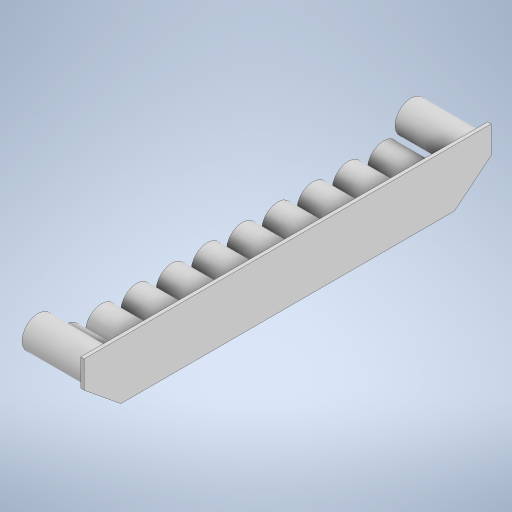
# Autodesk Inventor part: Enemy_Track_inertia
Saved by Autodesk Inventor 2024 (Build 280153000, 153)
## iProperties
Created: 2026-05-21
Part Number: Enemy_Track_inertia
Material: Generic
Document SubType Name: Modeling
Designer: warny
Density: 1 g/cm^3
Appearance: Default
Author: warny
Autodesk Inventor part; units mm, degrees
ref_plane "YZ Plane" through (0, 0, 0) normal (1, 0, 0) x (0, 1, 0)
ref_plane "XZ Plane" through (0, 0, 0) normal (0, 1, 0) x (-1, 0, 0)
ref_plane "XY Plane" through (0, 0, 0) normal (0, 0, 1) x (1, 0, 0)
sketch "Sketch1" plane through (0, 0, 0) normal (1, 0, 0) x (0, 1, 0)
  line L0 (66.79, 404) -> (66.79, -404)
  line L1 (66.79, -404) -> (12.72, -404)
  line L2 (12.72, -404) -> (-46.497, -331.3)
  line L3 (-46.497, -331.3) -> (-46.497, 331.3)
  line L4 (-46.497, 331.3) -> (12.72, 404)
  line L5 (12.72, 404) -> (66.79, 404)
  point P0 (0, 0)
  dimension "d0" = 331.3
  dimension "d1" = 331.3
  dimension "d2" = 46.497
  dimension "d3" = 46.497
  dimension "d4" = 12.72
  dimension "d5" = 12.72
  dimension "d6" = 404
  dimension "d7" = 404
  dimension "d8" = 66.79
  constraints: 12 end point, 1 parallel, 1 perpendicular, 1 vertical
  measures "d0" vertical distance of L3.end point (0, 0)
  measures "d1" vertical distance of point (0, 0) L2.end
  measures "d2" horizontal distance of L3.end point (0, 0)
  measures "d3" horizontal distance of L2.end point (0, 0)
  measures "d4" horizontal distance of L4.end point (0, 0)
  measures "d5" horizontal distance of L1.end point (0, 0)
  measures "d6" vertical distance of point (0, 0) L4.end
  measures "d7" vertical distance of point (0, 0) L1.end
  measures "d8" horizontal distance of L0.start point (0, 0)
extrude "Extrusion1" add sketch "Sketch1" along normal blind 66.5
sketch "Sketch2" plane through (0, 0, 0) normal (-1, 0, 0) x (0, 0, 1)
  line L0 (404, 66.79) -> (-404, 66.79) projected
  line L1 (-404, 66.79) -> (-404, 12.72) projected
  line L2 (-404, 12.72) -> (-331.3, -46.497) projected
  line L3 (331.3, -46.497) -> (404, 12.72) projected
  line L4 (404, 12.72) -> (404, 66.79) projected
  line L5 (404, 66.79) -> (-404, 66.79) projected
  line L6 (-404, 66.79) -> (-404, 12.72) projected
  line L7 (-404, 12.72) -> (-331.3, -46.497) projected
  line L8 (-331.3, -46.497) -> (331.3, -46.497) projected
  point P0 (0, 0)
extrude "Extrusion2" cut sketch "Sketch2" against normal blind 59.5
sketch "Sketch3" plane through (59.5, 0, 0) normal (-1, 0, 0) x (0, 0, 1)
  circle A0 centre (-370.6, 33.27) radius 31.6465
  circle A1 centre (-316, -13.01) radius 31.6465
  circle A2 centre (-246, -13.01) radius 31.6465
  circle A3 centre (-176, -13.01) radius 31.6465
  circle A4 centre (-106, -13.01) radius 31.6465
  circle A5 centre (-36, -13.01) radius 31.6465
  circle A6 centre (34, -13.01) radius 31.6465
  circle A7 centre (104, -13.01) radius 31.6465
  circle A8 centre (174, -13.01) radius 31.6465
  circle A9 centre (244, -13.01) radius 31.6465
  circle A10 centre (314, -13.01) radius 31.6465
  circle A11 centre (370, 33.27) radius 31.6465
  point P0 (0, 0)
  dimension "d13" = 33.27
  dimension "d14" = 33.27
  dimension "d15" = 370.6
  dimension "d16" = 370
  dimension "d17" = 316
  dimension "d18" = 13.01
  dimension "d19" = 70
  dimension "d20" = 70
  dimension "d21" = 70
  dimension "d22" = 70
  dimension "d23" = 70
  dimension "d24" = 70
  dimension "d25" = 70
  dimension "d26" = 70
  dimension "d27" = 70
  dimension "d28" = 13.01
  dimension "d29" = 13.01
  dimension "d30" = 13.01
  dimension "d31" = 13.01
  dimension "d32" = 13.01
  dimension "d33" = 13.01
  dimension "d34" = 13.01
  dimension "d35" = 13.01
  dimension "d36" = 13.01
  dimension "d37" = 63.293
  dimension "d38" = 63.293
  dimension "d39" = 63.293
  dimension "d40" = 63.293
  dimension "d41" = 63.293
  dimension "d42" = 63.293
  dimension "d43" = 63.293
  dimension "d44" = 63.293
  dimension "d45" = 63.293
  dimension "d46" = 63.293
  dimension "d47" = 63.293
  dimension "d48" = 63.293
  constraints: 12 centre point, 12 coincident
  measures "d13" vertical distance of point (-370.6, 33.27) point (0, 0)
  measures "d14" vertical distance of point (0, 0) point (370, 33.27)
  measures "d15" horizontal distance of point (-370.6, 33.27) point (0, 0)
  measures "d16" horizontal distance of point (0, 0) point (370, 33.27)
  measures "d17" horizontal distance of point (-316, -13.01) point (0, 0)
  measures "d18" vertical distance of point (-316, -13.01) point (0, 0)
  measures "d19" distance of point (-316, -13.01) point (-246, -13.01)
  measures "d20" distance of point (-246, -13.01) point (-176, -13.01)
  measures "d21" distance of point (-176, -13.01) point (-106, -13.01)
  measures "d22" distance of point (-106, -13.01) point (-36, -13.01)
  measures "d23" distance of point (-36, -13.01) point (34, -13.01)
  measures "d24" distance of point (34, -13.01) point (104, -13.01)
  measures "d25" distance of point (104, -13.01) point (174, -13.01)
  measures "d26" distance of point (174, -13.01) point (244, -13.01)
  measures "d27" distance of point (244, -13.01) point (314, -13.01)
  measures "d28" vertical distance of point (0, 0) point (-246, -13.01)
  measures "d29" vertical distance of point (0, 0) point (-176, -13.01)
  measures "d30" vertical distance of point (-106, -13.01) point (0, 0)
  measures "d31" vertical distance of point (0, 0) point (-36, -13.01)
  measures "d32" vertical distance of point (0, 0) point (34, -13.01)
  measures "d33" vertical distance of point (0, 0) point (104, -13.01)
  measures "d34" vertical distance of point (0, 0) point (174, -13.01)
  measures "d35" vertical distance of point (0, 0) point (244, -13.01)
  measures "d36" vertical distance of point (0, 0) point (314, -13.01)
  measures "d37" diameter of A0
  measures "d38" diameter of A1
  measures "d39" diameter of A2
  measures "d40" diameter of A3
  measures "d41" diameter of A4
  measures "d42" diameter of A5
  measures "d43" diameter of A6
  measures "d44" diameter of A7
  measures "d45" diameter of A8
  measures "d46" diameter of A9
  measures "d47" diameter of A10
  measures "d48" diameter of A11
extrude "Extrusion3" add sketch "Sketch3" along normal blind 119
sketch "Sketch4" plane through (-59.5, 33.27, -370.6) normal (-1, 0, 0) x (0, 0, 1)
  circle A0 centre (0, 0) radius 31.6465 projected
  point P0 (370.6, -33.27)
  constraints: 1 coincident
hole "Hole1" at (-59.5, 33.27, -370.6) direction (1, 0, 0) diameter 53 depth 119
pattern_sketch "Sketch Driven Pattern1" of "Hole1" from (59.5, 33.27, -370.6) copies at (59.5, 33.27, 370) at (59.5, -13.01, -316) at (59.5, -13.01, -246) at (59.5, -13.01, -176) at (59.5, -13.01, -106) at (59.5, -13.01, -36) at (59.5, -13.01, 34) at (59.5, -13.01, 104) at (59.5, -13.01, 174) at (59.5, -13.01, 244) at (59.5, -13.01, 314)
body "Solid1"
